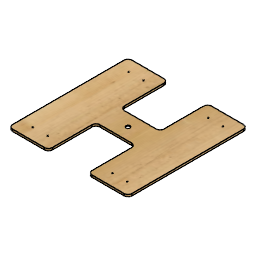
LB1 - Baseplate (Autodesk Fusion 360 design; units mm, degrees)
Autodesk Fusion 360 part; units mm, degrees
sketch "Sketch1" plane through (0, 0, 0) normal (0, 0, 1) x (1, 0, 0)
  line L0 (40, 31) -> (-40, 31)
  line L1 (-40, -31) -> (40, -31)
  line L2 (50, 31) -> (-50, -31) construction
  line L3 (-50, 31) -> (50, -31) construction
  line L4 (151, 31) -> (151, 141)
  line L5 (141, 151) -> (60, 151)
  line L6 (50, 141) -> (50, 41)
  line L7 (151, -31) -> (151, -141)
  line L8 (141, -151) -> (60, -151)
  line L9 (50, -141) -> (50, -41)
  line L10 (151, -31) -> (151, 31)
  line L11 (0, 0) -> (0, 31) construction
  line L12 (-141, 151) -> (-60, 151)
  line L13 (-50, 141) -> (-50, 41)
  line L14 (-151, 31) -> (-151, 141)
  line L15 (-151, -31) -> (-151, 31)
  line L16 (-141, -151) -> (-60, -151)
  line L17 (-50, -141) -> (-50, -41)
  line L18 (-151, -31) -> (-151, -141)
  circle A0 centre (0, 0) radius 5
  arc A1 (-141, 151) -> (-151, 141) centre (-141, 141) ccw
  arc A2 (-50, 141) -> (-60, 151) centre (-60, 141) ccw
  arc A3 (60, 151) -> (50, 141) centre (60, 141) ccw
  arc A4 (151, 141) -> (141, 151) centre (141, 141) ccw
  arc A5 (-151, -141) -> (-141, -151) centre (-141, -141) ccw
  arc A6 (-60, -151) -> (-50, -141) centre (-60, -141) ccw
  arc A7 (50, -141) -> (60, -151) centre (60, -141) ccw
  arc A8 (141, -151) -> (151, -141) centre (141, -141) ccw
  arc A9 (-40, -31) -> (-50, -41) centre (-40, -41) ccw
  arc A10 (50, -41) -> (40, -31) centre (40, -41) ccw
  arc A11 (40, 31) -> (50, 41) centre (40, 41) ccw
  arc A12 (-50, 41) -> (-40, 31) centre (-40, 41) ccw
  line L19 (100.5, -151) -> (100.5, -121) construction
  line L20 (119.25, -121) -> (81.75, -121) construction
  circle A13 centre (119.25, -121) radius 1.5
  circle A14 centre (81.75, -121) radius 1.5
  line L21 (151, 0) -> (100, 0) construction
  circle A15 centre (81.75, 121) radius 1.5
  circle A16 centre (119.25, 121) radius 1.5
  line L22 (0, -150) -> (0, -125) construction
  circle A17 centre (-81.75, -121) radius 1.5
  circle A18 centre (-119.25, -121) radius 1.5
  circle A19 centre (-81.75, 121) radius 1.5
  circle A20 centre (-119.25, 121) radius 1.5
  point P0 (50, 151)
  point P1 (50, -151)
  dimension "d1" = 100
  dimension "d2" = 62
  dimension "d3" = 101
  dimension "d4" = 120
  dimension "d5" = 101
  dimension "d6" = 120
  dimension "d9" = 10
  dimension "d10" = 10
  dimension "d11" = 30
  dimension "d12" = 18.75
  dimension "d13" = 37.5
  dimension "d14" = 3
  dimension "d15" = 3
  dimension "d21" = 51
  dimension "d22" = 25
  dimension "d23" = 125
  constraint horizontal L0
  constraint parallel L0 L1
  constraint coincident L2 L11.start
  constraint coincident L3 L11.start
  constraint coincident L11.start A0.centre
  constraint vertical L4
  constraint horizontal L5
  constraint vertical L6
  constraint vertical L7
  constraint horizontal L8
  constraint vertical L9
  constraint symmetric L4.start L11 L14.start
  constraint symmetric L7.start L11 L15.start
  constraint tangent L12 A1
  constraint tangent L14 A1
  constraint tangent L12 A2
  constraint tangent L13 A2
  constraint equal A1 A2
  constraint coincident P0 L5
  constraint coincident P0 L6
  constraint tangent L5 A3
  constraint tangent L6 A3
  constraint equal A1 A3
  constraint tangent L4 A4
  constraint tangent L5 A4
  constraint equal A1 A4
  constraint tangent L16 A5
  constraint tangent L18 A5
  constraint equal A1 A5
  constraint tangent L16 A6
  constraint tangent L17 A6
  constraint equal A1 A6
  constraint coincident P1 L8
  constraint coincident P1 L9
  constraint tangent L8 A7
  constraint tangent L9 A7
  constraint equal A1 A7
  constraint tangent L7 A8
  constraint tangent L8 A8
  constraint equal A1 A8
  constraint coincident L2.end L1
  constraint tangent L1 A9
  constraint tangent L17 A9
  constraint equal A1 A9
  constraint coincident L3.end L1
  constraint coincident L3.end L9
  constraint tangent L1 A10
  constraint tangent L9 A10
  constraint equal A1 A10
  constraint coincident L0 L11.end
  constraint coincident L2.start L6
  constraint coincident L2.start L0
  constraint tangent L6 A11
  constraint tangent L0 A11
  constraint equal A1 A11
  constraint coincident L3.start L0
  constraint tangent L13 A12
  constraint tangent L0 A12
  constraint equal A1 A12
  constraint midpoint L8 L19.start
  constraint perpendicular L8 L19
  constraint coincident L20.start A13.centre
  constraint coincident L20.end A14.centre
  constraint midpoint L10 L21.start
  constraint perpendicular L10 L21
  constraint symmetric A13 L21 A16
  constraint symmetric A14 L21 A15
  constraint vertical L22
  constraint symmetric A13 L22 A18
  constraint symmetric A14 L22 A17
  constraint symmetric A15 L22 A19
  constraint symmetric A16 L22 A20
  constraint parallel L14 L18
  constraint parallel L4 L17
  constraint parallel L1 L12
  constraint parallel L7 L14
  constraint parallel L4 L10
  constraint parallel L4 L13
  constraint parallel L4 L15
  constraint parallel L5 L16
  constraint collinear L5 L12
  constraint collinear L6 L9
  constraint collinear L8 L16
  constraint collinear L11 L22
  constraint collinear L13 L17
  constraint horizontal L20
  constraint vertical L2.end L17.start
  constraint vertical L3.start L17.start
  constraint horizontal L2.start L4.start
  constraint horizontal L19.end A18.centre
  constraint horizontal L11.start L21.end
  measures "d1" distance of L2.end L3.end
  measures "d2" distance of L3.start L2.end
  measures "d3" distance of L2.start L4.start
  measures "d4" distance of L2.start P0
  measures "d5" distance of L3.end L7.start
  measures "d6" distance of L3.end P1
  measures "d9" diameter of A0
  measures "d10" radius of A1
  measures "d11" distance of L19.start L19.end
  measures "d12" distance of L19.end L20.start
  measures "d13" distance of L20.start L20.end
  measures "d14" diameter of A13
  measures "d15" diameter of A14
  measures "d21" distance of L4 L21.end
  measures "d22" vertical distance of L22.start L22.end
  measures "d23" vertical distance of L11.start L22.end
extrude "Extrude1" add sketch "Sketch1" along normal blind 30.6
chamfer "Chamfer1" distance 5.2024 angle 41 1 edges at (-4.6616, 1.8081, 0) measured on face at (4.9938, -0.2492, 20.4)
extrude "Extrude2" cut 1 faces at (-96.5316, 12.7276, 30.6) along direction (0, 0, -1) blind 25.4
equation "d7 = 5.2 mm + 1 in"
equation "d12 = ( 37.5 / 2 ) * 1 mm"
